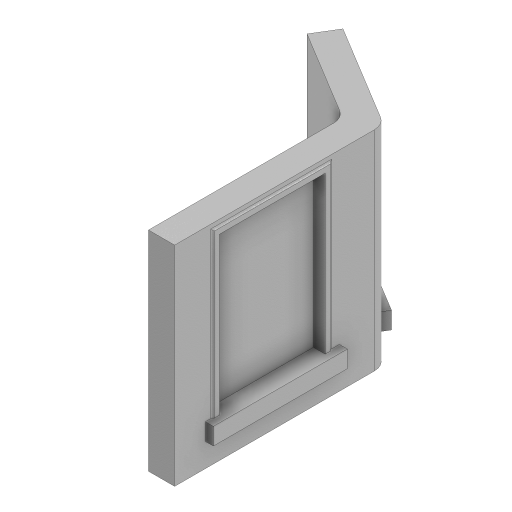
# Autodesk Inventor part: wall
Saved by Autodesk Inventor 2023 (Build 270158000, 158)
## iProperties
Created: 2022-08-08
Part Number: wall
Material: Generic
Document SubType Name: Modeling
Designer: Derm
Density: 1 g/cm^3
Appearance: Smooth - Beige
Author: Derm
Autodesk Inventor part; units mm, degrees
ref_plane "YZ Plane" through (0, 0, 0) normal (1, 0, 0) x (0, 1, 0)
ref_plane "XZ Plane" through (0, 0, 0) normal (0, 1, 0) x (-1, 0, 0)
ref_plane "XY Plane" through (0, 0, 0) normal (0, 0, 1) x (1, 0, 0)
sketch "Sketch1" plane through (0, 0, 0) normal (0, 0, 1) x (1, 0, 0)
  line L0 (0, 0) -> (500, 0)
  line L1 (500, 0) -> (500, 4000)
  line L2 (500, 4000) -> (0, 4000)
  line L3 (0, 4000) -> (0, 0)
  point P0 (250, 0)
  dimension "d0" = 500
  dimension "d1" = 4000
  constraints: 8 end point, 2 parallel, 1 horizontal, 1 midpoint, 1 perpendicular
  measures "d0" distance between parallel lines of L1 L3
  measures "d1" distance from line of point (250, 0) L2
extrude "Extrusion1" add sketch "Sketch1" along normal mid plane 3000
sketch "Sketch2" plane through (0, 4000, 1500) normal (0, 1, 0) x (1, 0, 0)
  line L0 (0, 3000) -> (0, 0)
  line L1 (500, 0) -> (0, 0)
  line L2 (500, 3000) -> (500, 0)
  line L3 (0, 3000) -> (500, 3000)
  line L4 (500, 3000) -> (-1473.742944, 4196.058603)
  line L5 (0, 2718.352049) -> (-1732.870154, 3768.445356)
  line L6 (-1473.742944, 4196.058603) -> (-1732.870154, 3768.445356)
  point P0 (0, 1500)
  dimension "d18" = 500
  constraints: 6 end point, 1 parallel, 1 perpendicular, 1 point on line
  measures "d18" distance between parallel lines of L4 L5
extrude "Extrusion4" add sketch "Sketch2" against normal up to surface (4000 mm away) contours L0 L5 L6 L4 L3
fillet "Fillet2" radius 304.8 2 edges at (500, 2000, -1500) (0, 2000, -1218.352)
fillet "Fillet3" [suppressed]
fillet "Fillet4" [suppressed]
sketch "Sketch4" plane through (0, 0, 1500) normal (0, 0, 1) x (1, 0, 0)
  line L0 (0, 4000) -> (0, 0) projected
  line L1 (0, 0) -> (500, 0) projected
  line L2 (500, 0) -> (500, 4000) projected
  line L3 (500, 4000) -> (0, 4000) projected
extrude "Extrusion5" add sketch "Sketch4" along normal blind 1000
ref_plane "Work Plane3" through (0, 776.2875, 2500) normal (0, -1, 0) x (1, 0, 0)
sketch "Sketch5" plane through (0, 776.2875, 2500) normal (0, 1, 0) x (1, 0, 0)
  arc A0 (500, 3828.307409) -> (353.163947, 4088.980444) centre (195.2, 3828.307409) ccw
  line L0 (500, 0) -> (500, 3828.307409)
  line L1 (0, 0) -> (500, 0)
  line L2 (0, 3546.659458) -> (0, 0)
  arc A1 (0, 3546.659458) -> (-146.836053, 3807.332493) centre (-304.8, 3546.659458) ccw
  line L3 (-1732.870154, 4768.445356) -> (-146.836053, 3807.332493)
  line L4 (-1473.742944, 5196.058603) -> (-1732.870154, 4768.445356)
  line L5 (353.163947, 4088.980444) -> (-1473.742944, 5196.058603)
  line L6 (500, 835.948332) -> (300.402706, 835.948332)
  line L7 (300.402706, 835.948332) -> (300.402706, 2857.961935)
  line L8 (300.402706, 2857.961935) -> (500, 2857.961935)
  line L9 (141.793524, 4217.067748) -> (20.592459, 4017.061037)
  line L10 (20.592459, 4017.061037) -> (-946.13138, 4602.881175)
  line L11 (-946.13138, 4602.881175) -> (-824.930314, 4802.887887)
  point P0 (0, 2500)
  constraints: 12 end point, 4 point on line, 3 perpendicular, 2 parallel, 1 horizontal
extrude "Extrusion6" cut sketch "Sketch5" along normal blind 3000 contours L0 L6 L7 L8 | L9 L10 L11 L5
sketch "Sketch6" plane through (500, 0, -1328.307409) normal (1, 0, 0) x (0, 0, -1)
  line L0 (-970.345474, 776.2875) -> (-2992.359077, 776.2875)
  line L1 (-970.345474, 776.2875) -> (-970.345474, 3776.2875)
  line L2 (-970.345474, 3776.2875) -> (-2992.359077, 3776.2875)
  line L3 (-2992.359077, 776.2875) -> (-2992.359077, 3776.2875)
  line L4 (-3093.959077, 3877.8875) -> (-868.745474, 3877.8875)
  line L5 (-868.745474, 3877.8875) -> (-868.745474, 674.6875)
  line L6 (-868.745474, 674.6875) -> (-3093.959077, 674.6875)
  line L7 (-3093.959077, 674.6875) -> (-3093.959077, 3877.8875)
  point P0 (-1328.307409, 0)
  dimension "d29" = 101.6
  constraints: 8 end point, 3 other
  measures "d29" distance between parallel lines of L2 L4
extrude "Extrusion7" add sketch "Sketch6" along normal blind 25.4
sketch "Sketch7" plane through (-1473.742944, 0, -2696.058603) normal (0.5182544, 0, -0.8552265) x (-0.8552265, 0, -0.5182544)
  line L0 (-758.644212, 776.2875) -> (-1889.015927, 776.2875)
  line L1 (-758.644212, 776.2875) -> (-758.644212, 3776.2875)
  line L2 (-758.644212, 3776.2875) -> (-1889.015927, 3776.2875)
  line L3 (-1889.015927, 776.2875) -> (-1889.015927, 3776.2875)
  line L4 (-1990.615927, 3877.8875) -> (-657.044212, 3877.8875)
  line L5 (-657.044212, 3877.8875) -> (-657.044212, 674.6875)
  line L6 (-657.044212, 674.6875) -> (-1990.615927, 674.6875)
  line L7 (-1990.615927, 674.6875) -> (-1990.615927, 3877.8875)
  point P0 (-2657.628299, 0)
  dimension "d32" = 101.6
  constraints: 8 end point, 3 other
  measures "d32" distance between parallel lines of L2 L4
extrude "Extrusion8" add sketch "Sketch7" along normal blind 25.4
fillet "Fillet5" radius 50.8 8 edges at (500, 674.6875, 653.0449) (500, 2276.2875, -459.5619) (500, 3877.8875, 653.0449) (500, 2276.2875, 1765.6517) (-911.8213, 2276.2875, -2355.5425) (-341.5684, 674.6875, -2009.9778) (228.6845, 2276.2875, -1664.4131) (-341.5684, 3877.8875, -2009.9778)
sketch "Sketch8" plane through (500, 0, -1328.307409) normal (1, 0, 0) x (0, 0, -1)
  line L0 (-3093.959077, 674.6875) -> (-868.745474, 674.6875)
  line L1 (-868.745474, 674.6875) -> (-868.745474, 3877.8875)
  line L2 (-868.745474, 3877.8875) -> (-3093.959077, 3877.8875)
  line L3 (-3093.959077, 3877.8875) -> (-3093.959077, 674.6875)
  line L4 (-970.345474, 3776.2875) -> (-970.345474, 776.2875)
  line L5 (-970.345474, 776.2875) -> (-2992.359077, 776.2875)
  line L6 (-2992.359077, 776.2875) -> (-2992.359077, 3776.2875)
  line L7 (-2992.359077, 3776.2875) -> (-970.345474, 3776.2875)
  line L8 (-3238.573166, 776.2875) -> (-674.319307, 776.2875)
  line L9 (-674.319307, 776.2875) -> (-674.319307, 449.778373)
  line L10 (-674.319307, 449.778373) -> (-3238.573166, 449.778373)
  line L11 (-3238.573166, 449.778373) -> (-3238.573166, 776.2875)
  point P0 (-1328.307409, 0)
  point P1 (-3093.959077, 776.2875)
  point P2 (-868.745474, 776.2875)
  point P3 (-970.345474, 776.2875)
  point P4 (-2992.359077, 776.2875)
  constraints: 8 end point, 2 parallel, 1 horizontal, 1 perpendicular
extrude "Extrusion9" add sketch "Sketch8" along normal blind 152.4 contours L3 L8 L5 L1 L0 | L0 L1 L8 L9 L10 L11 L3
sketch "Sketch9" plane through (-1473.742944, 0, -2696.058603) normal (0.5182544, 0, -0.8552265) x (-0.8552265, 0, -0.5182544)
  line L0 (-2136.167325, 0) -> (-2136.167325, 4000)
  line L1 (-2136.167325, 0) -> (0, 0)
  line L2 (0, 4000) -> (0, 0)
  line L3 (-2136.167325, 4000) -> (0, 4000)
  line L4 (-2034.610018, 3921.881591) -> (-2034.610018, 630.693409)
  line L5 (-613.050122, 3921.881591) -> (-2034.610018, 3921.881591)
  line L6 (-613.050122, 630.693409) -> (-613.050122, 3921.881591)
  line L7 (-2034.610018, 630.693409) -> (-613.050122, 630.693409)
  line L8 (-2876.645839, 776.2875) -> (-4205.581737, 776.2875)
  line L9 (-4205.581737, 776.2875) -> (-4205.581737, 449.778373)
  line L10 (-4205.581737, 449.778373) -> (-2876.645839, 449.778373)
  line L11 (-2876.645839, 449.778373) -> (-2876.645839, 776.2875)
  line L12 (-2136.167325, 776.2875) -> (-546.983817, 776.2875)
  line L13 (-546.983817, 776.2875) -> (-546.983817, 449.778373)
  line L14 (-546.983817, 449.778373) -> (-2136.167325, 449.778373)
  line L15 (-2136.167325, 449.778373) -> (-2136.167325, 776.2875)
  point P0 (-2657.628299, 0)
  point P1 (-2136.167325, 449.778373)
  constraints: 8 end point, 2 parallel, 1 horizontal, 1 perpendicular, 1 point on line
extrude "Extrusion10" add sketch "Sketch9" along normal blind 152.4 contours L0 L12 L4 L7 L6 L13 L14 | L12 L6 L7 L4
body "Solid1"
